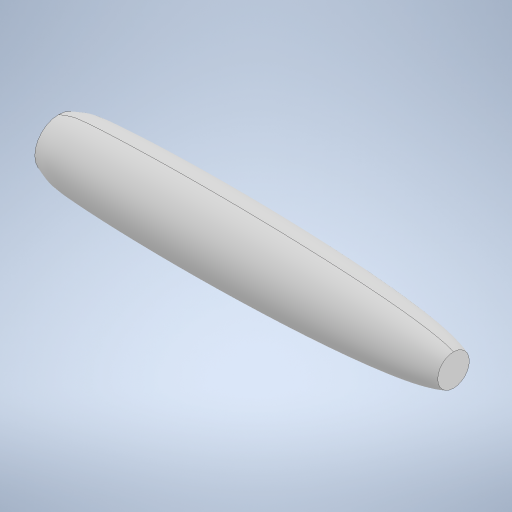
# Autodesk Inventor part: parker-penw
Saved by Autodesk Inventor 2023 (Build 270158030, 158C)
## iProperties
Created: 2024-03-10
Part Number: parker-penw
Material: Generic
Document SubType Name: Modeling
Designer: Imogen Heard
Density: 1 g/cm^3
Appearance: Default
Author: Imogen Heard
Autodesk Inventor part; units mm, degrees
ref_plane "YZ Plane" through (0, 0, 0) normal (1, 0, 0) x (0, 1, 0)
ref_plane "XZ Plane" through (0, 0, 0) normal (0, 1, 0) x (-1, 0, 0)
ref_plane "XY Plane" through (0, 0, 0) normal (0, 0, 1) x (1, 0, 0)
sketch "Sketch3" plane through (0, 0, 0) normal (0, 0, 1) x (1, 0, 0)
  line L0 (50, 4) -> (50, 0)
  line L1 (50, 0) -> (-50, 0)
  line L2 (-50, 0) -> (-50, 6)
  line L3 (-50, 6) -> (-46.4301, 7.4519) construction
  line L4 (40.4256, 8.2824) -> (50, 4) construction
  spline S0 degree 4 poles (-50, 6) (-46.4301, 7.4519) (-38.6817, 8.2824) (-11.9355, 9.6224) (40.4256, 8.2824) (50, 4) knots 1 1 1 1 1 1.137034 2 2 2 2 2
  line L5 (-46.4301, 7.4519) -> (-38.6817, 8.2824) construction
  line L6 (-38.6817, 8.2824) -> (-11.9355, 9.6224) construction
  line L7 (-11.9355, 9.6224) -> (40.4256, 8.2824) construction
  point P0 (0, 0)
  dimension "d1" = 100
  dimension "d2" = 6
  dimension "d3" = 4
  dimension "d10" = 50
  constraints: 6 end point, 1 horizontal alignment, 1 parallel, 3 other
  measures "d1" distance between parallel lines of L0 L2
  measures "d2" vertical distance of L2.end point (0, 0)
  measures "d3" vertical distance of point (0, 0) L0.start
  measures "d10" distance of point (0, 0) L1.end
revolve "Revolution1" add sketch "Sketch3" angle 360 about axis through (50, 0, 0) along (-1, 0, 0)
equation "\"d10\" = 0.5 * d1"
body "Solid1"
